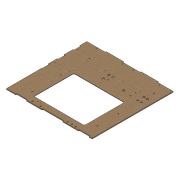
# Autodesk Inventor part: Lateral Izquierdo Carcasa
Saved by Autodesk Inventor 2020 (Build 240168000, 168)
## iProperties
Created: 2020-06-08
Part Number: Lateral Izquierdo Carcasa
Material: MDF Tablero de fibras de densidad media
Document SubType Name: Modelado
Designer: Pipi
Density: 0.8 g/cm^3
Appearance: Cartón - Ondulado
Mass: 1381.88 g
Surface Area: 4222.27 cm^2
Volume: 1727.35 cm^3
Sheet Metal Rule: Default
Author: Pipi
Autodesk Inventor part; units mm, degrees
ref_plane "YZ Plane" through (0, 0, 0) normal (1, 0, 0) x (0, 1, 0)
ref_plane "XZ Plane" through (0, 0, 0) normal (0, 1, 0) x (-1, 0, 0)
ref_plane "XY Plane" through (0, 0, 0) normal (0, 0, 1) x (1, 0, 0)
sketch "Boceto1" plane through (0, 0, 0) normal (0, 1, 0) x (-1, 0, 0)
  line L0 (67.9623, 11.1833) -> (67.9623, -453.8167)
  line L1 (435.9623, -258.8167) -> (159.9623, -258.8167)
  line L2 (152.9623, -251.8167) -> (152.9623, -35.8167)
  line L3 (159.9623, -28.8167) -> (435.9623, -28.8167)
  line L4 (442.9623, -35.8167) -> (442.9623, -251.8167)
  arc A0 (435.9623, -258.8167) -> (442.9623, -251.8167) centre (435.9623, -251.8167) ccw
  arc A1 (442.9623, -35.8167) -> (435.9623, -28.8167) centre (435.9623, -35.8167) ccw
  arc A2 (159.9623, -28.8167) -> (152.9623, -35.8167) centre (159.9623, -35.8167) ccw
  arc A3 (152.9623, -251.8167) -> (159.9623, -258.8167) centre (159.9623, -251.8167) ccw
  line L5 (449.9623, -251.8167) -> (449.9623, -35.8167)
  line L6 (435.9623, -21.8167) -> (159.9623, -21.8167)
  line L7 (145.9623, -35.8167) -> (145.9623, -251.8167)
  line L8 (159.9623, -265.8167) -> (435.9623, -265.8167)
  line L9 (159.9623, -265.8167) -> (152.9623, -265.8167)
  line L10 (145.9623, -258.8167) -> (145.9623, -251.8167)
  line L11 (159.9623, -21.8167) -> (152.9623, -21.8167)
  line L12 (145.9623, -28.8167) -> (145.9623, -35.8167)
  line L13 (435.9623, -21.8167) -> (442.9623, -21.8167)
  line L14 (449.9623, -28.8167) -> (449.9623, -35.8167)
  line L15 (449.9623, -251.8167) -> (449.9623, -258.8167)
  line L16 (442.9623, -265.8167) -> (435.9623, -265.8167)
  arc A4 (449.9623, -28.8167) -> (442.9623, -21.8167) centre (442.9623, -28.8167) ccw
  arc A5 (442.9623, -265.8167) -> (449.9623, -258.8167) centre (442.9623, -258.8167) ccw
  arc A6 (145.9623, -258.8167) -> (152.9623, -265.8167) centre (152.9623, -258.8167) ccw
  arc A7 (152.9623, -21.8167) -> (145.9623, -28.8167) centre (152.9623, -28.8167) ccw
  line L17 (557.9623, -453.8167) -> (457.9623, -453.8167)
  line L18 (457.9623, -453.8167) -> (457.9623, -459.3167)
  line L19 (457.9623, -459.3167) -> (357.9623, -459.3167)
  line L20 (357.9623, -459.3167) -> (357.9623, -453.8167)
  line L21 (357.9623, -453.8167) -> (257.9623, -453.8167)
  line L22 (257.9623, -453.8167) -> (257.9623, -459.3167)
  line L23 (257.9623, -459.3167) -> (157.9623, -459.3167)
  line L24 (157.9623, -459.3167) -> (157.9623, -453.8167)
  line L25 (157.9623, -453.8167) -> (67.9623, -453.8167)
  line L26 (157.9623, -459.3167) -> (257.9623, -459.3167)
  line L27 (357.9623, -459.3167) -> (457.9623, -459.3167)
  line L28 (355.9623, 11.1833) -> (355.9623, 5.6833)
  line L29 (355.9623, 5.6833) -> (235.9623, 5.6833)
  line L30 (235.9623, 5.6833) -> (235.9623, 11.1833)
  line L31 (67.9623, 11.1833) -> (85.9623, 11.1833)
  circle A8 centre (112.9623, -63.8167) radius 3
  circle A9 centre (112.9623, -183.8167) radius 3
  line L32 (67.9623, 11.1833) -> (85.9623, 11.1833)
  line L33 (87.9623, 5.6833) -> (87.9623, -422.8167)
  line L34 (87.9623, -422.8167) -> (137.9623, -422.8167)
  line L35 (137.9623, -422.8167) -> (137.9623, 5.6833)
  circle A10 centre (112.9623, -388.3167) radius 3
  line L36 (557.9623, 11.1833) -> (560.4623, 11.1833)
  line L37 (560.4623, 11.1833) -> (560.4623, -193.8167)
  line L38 (560.4623, -193.8167) -> (557.9623, -193.8167)
  line L39 (557.9623, -193.8167) -> (557.9623, -233.8168)
  line L40 (557.9623, -233.8168) -> (563.4623, -233.8168)
  line L41 (563.4623, -233.8168) -> (563.4623, -283.8168)
  line L42 (563.4623, -283.8168) -> (557.9623, -283.8168)
  line L43 (557.9623, -283.8168) -> (557.9623, -323.8168)
  line L44 (557.9623, -323.8168) -> (563.4623, -323.8168)
  line L45 (563.4623, -323.8168) -> (563.4623, -373.8168)
  line L46 (563.4623, -373.8168) -> (557.9623, -373.8168)
  line L47 (557.9623, -373.8168) -> (557.9623, -413.8168)
  line L48 (557.9623, -413.8168) -> (563.4623, -413.8168)
  line L49 (563.4623, -413.8168) -> (563.4623, -453.8167)
  line L50 (426.4606, 11.1833) -> (362.9606, 11.1833)
  arc A11 (376.2623, 2.6833) -> (371.2623, 2.6833) centre (373.7623, 2.6833) ccw
  arc A12 (399.7123, 1.6833) -> (394.7123, 1.6833) centre (397.2123, 1.6833) ccw
  arc A13 (424.1623, 2.6833) -> (419.1623, 2.6833) centre (421.6623, 2.6833) ccw
  line L51 (371.2623, 2.6833) -> (371.2623, -1.3167)
  line L52 (376.2623, 2.6833) -> (376.2623, -1.3167)
  arc A14 (371.2623, -1.3167) -> (376.2623, -1.3167) centre (373.7623, -1.3167) ccw
  line L53 (419.1623, 2.6833) -> (419.1623, -1.3167)
  line L54 (424.1623, 2.6833) -> (424.1623, -1.3167)
  arc A15 (419.1623, -1.3167) -> (424.1623, -1.3167) centre (421.6623, -1.3167) ccw
  line L55 (394.7123, 1.6833) -> (394.7123, -1.8167)
  line L56 (399.7123, 1.6833) -> (399.7123, -1.8167)
  arc A16 (394.7123, -1.8167) -> (399.7123, -1.8167) centre (397.2123, -1.8167) ccw
  line L57 (162.9623, 11.1833) -> (226.4623, 11.1833)
  arc A17 (221.6623, 2.6833) -> (216.6623, 2.6833) centre (219.1623, 2.6833) ccw
  arc A18 (197.2123, 1.6833) -> (192.2123, 1.6833) centre (194.7123, 1.6833) ccw
  arc A19 (173.7623, 2.6833) -> (168.7623, 2.6833) centre (171.2623, 2.6833) ccw
  line L58 (221.6623, 2.6833) -> (221.6623, -1.3167)
  line L59 (216.6623, 2.6833) -> (216.6623, -1.3167)
  arc A20 (216.6623, -1.3167) -> (221.6623, -1.3167) centre (219.1623, -1.3167) ccw
  line L60 (173.7623, 2.6833) -> (173.7623, -1.3167)
  line L61 (168.7623, 2.6833) -> (168.7623, -1.3167)
  arc A21 (168.7623, -1.3167) -> (173.7623, -1.3167) centre (171.2623, -1.3167) ccw
  line L62 (197.2123, 1.6833) -> (197.2123, -1.8167)
  line L63 (192.2123, 1.6833) -> (192.2123, -1.8167)
  arc A22 (192.2123, -1.8167) -> (197.2123, -1.8167) centre (194.7123, -1.8167) ccw
  line L64 (563.4623, -453.8167) -> (557.9623, -453.8167)
  circle A23 centre (498.4623, -445.3167) radius 2
  circle A24 centre (348.4623, -445.3167) radius 2
  circle A25 centre (137.9623, -445.3167) radius 2
  circle A26 centre (287.9623, -445.3167) radius 2
  circle A27 centre (550.2473, -388.8167) radius 2
  circle A28 centre (550.2473, -258.8167) radius 2
  circle A29 centre (77.6773, -448.8167) radius 2
  line L65 (355.9623, 11.1833) -> (445.9623, 11.1833)
  line L66 (445.9623, 11.1833) -> (445.9623, 5.6833)
  line L67 (445.9623, 5.6833) -> (505.9623, 5.6833)
  line L68 (505.9623, 5.6833) -> (505.9623, 11.1833)
  line L69 (557.9623, 11.1833) -> (505.9623, 11.1833)
  line L70 (445.9623, 11.1833) -> (355.9623, 11.1833)
  line L71 (235.9623, 11.1833) -> (145.9623, 11.1833)
  line L72 (145.9623, 11.1833) -> (145.9623, 5.6833)
  line L73 (145.9623, 5.6833) -> (85.9623, 5.6833)
  line L74 (85.9623, 5.6833) -> (85.9623, 11.1833)
  line L75 (235.9623, 11.1833) -> (145.9623, 11.1833)
  line L76 (85.9623, 11.1833) -> (67.9623, 11.1833)
  circle A30 centre (403.7123, -13.8167) radius 1.5
  circle A31 centre (390.7123, -13.8167) radius 1.5
  point P0 (145.9623, -21.8167)
  point P1 (449.9623, -21.8167)
  point P2 (449.9623, -265.8167)
  point P3 (0, 0)
  point P4 (0, 0)
  point P5 (426.4606, 11.1833)
  point P6 (362.9606, 11.1833)
  dimension "d217" = 85
  dimension "d219" = 7
  dimension "d232" = 230
  dimension "d233" = 7
  dimension "d234" = 7
  dimension "d236" = 100
  dimension "d237" = 100
  dimension "d238" = 100
  dimension "d239" = 100
  dimension "d241" = 465
  dimension "d288" = 202
  dimension "d289" = 5.5
  dimension "d292" = 168
  dimension "d312" = 6
  dimension "d314" = 6
  dimension "d319" = 120
  dimension "d325" = 50
  dimension "d326" = 25
  dimension "d327" = 25
  dimension "d328" = 6
  dimension "d329" = 25
  dimension "d332" = 34.5
  dimension "d333" = 2.5
  dimension "d334" = 205
  dimension "d336" = 27.5
  dimension "d337" = 7
  dimension "d338" = 7
  dimension "d339" = 5.5
  dimension "d342" = 40.0001
  dimension "d344" = 465
  dimension "d346" = 2.5
  dimension "d347" = 50
  dimension "d348" = 40
  dimension "d349" = 50
  dimension "d350" = 40
  dimension "d384" = 5
  dimension "d385" = 5
  dimension "d386" = 5
  dimension "d394" = 4
  dimension "d395" = 4
  dimension "d396" = 4
  dimension "d397" = 4
  dimension "d398" = 3.5
  dimension "d399" = 3.5
  dimension "d404" = 15.3
  dimension "d405" = 120
  dimension "d406" = 495.5
  dimension "d420" = 5.5
  dimension "d423" = 4
  dimension "d424" = 65
  dimension "d425" = 8.5
  dimension "d426" = 4
  dimension "d427" = 150
  dimension "d428" = 4
  dimension "d429" = 8.5
  dimension "d430" = 70
  dimension "d431" = 4
  dimension "d432" = 150
  dimension "d435" = 4
  dimension "d436" = 4
  dimension "d437" = 7.715
  dimension "d438" = 7.715
  dimension "d439" = 65
  dimension "d440" = 130
  constraints: 154 end point, 44 perpendicular, 40 point on circle, 32 centre point, 25 tangent, 19 point on line, 7 horizontal, 6 equal radius, 4 parallel, 3 collinear, 2 vertical
  measures "d217" distance between parallel lines of L0 L2
  measures "d219" radius of A0
  measures "d232" distance between parallel lines of L1 L3
  measures "d233" distance between parallel lines of L4 L5
  measures "d234" radius of A4
  measures "d236" distance of L17.start L17.end
  measures "d237" distance of L18.end L19.end
  measures "d238" distance of L20.end L21.end
  measures "d239" distance of L23.end L22.end
  measures "d241" distance of L0.start L0.end
  measures "d288" distance of L36.start L28.start
  measures "d289" distance of L28.start L28.end
  measures "d292" distance of L30.end L0.start
  measures "d312" diameter of A8
  measures "d314" diameter of A9
  measures "d319" distance of A9.centre A8.centre
  measures "d325" distance of L33.end L34.end
  measures "d326" distance from line of L35 A8.centre
  measures "d327" distance from line of L35 A9.centre
  measures "d328" diameter of A10
  measures "d329" distance from line of L35 A10.centre
  measures "d332" distance from line of L34 A10.centre
  measures "d333" distance of L36.start L36.end
  measures "d334" distance of L36.end L37.end
  measures "d336" distance between parallel lines of L29 L6
  measures "d337" distance between parallel lines of L6 L3
  measures "d338" distance between parallel lines of L1 L8
  measures "d339" distance of L17.start L49.end
  measures "d342" distance of L38.end L39.end
  measures "d344" distance from line of L36.end L17
  measures "d346" distance of L38.end L37.end
  measures "d347" distance of L40.end L41.end
  measures "d348" distance of L42.end L43.end
  measures "d349" distance of L44.end L45.end
  measures "d350" distance of L46.end L47.end
  measures "d384" diameter of A11
  measures "d385" diameter of A12
  measures "d386" diameter of A13
  measures "d394" distance of L51.start L51.end
  measures "d395" distance of L52.start L52.end
  measures "d396" distance of L53.start L53.end
  measures "d397" distance of L54.start L54.end
  measures "d398" distance of L55.start L55.end
  measures "d399" distance of L56.start L56.end
  measures "d404" distance between parallel lines of L51 L28
  measures "d405" distance of L28.end L29.end
  measures "d406" distance between parallel lines of L0 L49
  measures "d420" distance between parallel lines of L43 L41
  measures "d423" diameter of A23
  measures "d424" distance from line of L49 A23.centre
  measures "d425" distance from line of L17 A23.centre
  measures "d426" diameter of A24
  measures "d427" distance of A24.centre A23.centre
  measures "d428" diameter of A25
  measures "d429" distance from line of L25 A25.centre
  measures "d430" distance from line of L0 A25.centre
  measures "d431" diameter of A26
  measures "d432" distance of A25.centre A26.centre
  measures "d435" diameter of A27
  measures "d436" diameter of A28
  measures "d437" distance from line of L47 A27.centre
  measures "d438" distance from line of L47 A28.centre
  measures "d439" distance from line of L17 A27.centre
  measures "d440" distance of A28.centre A27.centre
extrude "Extrusión1" add sketch "Boceto1" against normal blind 5.5 contours L31 L74 L73 L33 L34 L35 L72 L71 L57 L30 L29 L28 L65 L50 L66 L67 L68 L69 L36 L37 L38 L39 L40 L41 L42 L43 L44 L45 L46 L47 L48 L49 L64 L17 L18 L19 L20 L21 L22 L23 L24 L25 L0 | L73 L35 L34 L33 | L56 A16 L55 A12
extrude "Extrusión4" add sketch "Boceto1" against normal blind 2.5 contours L15 A5 L16 L8 L9 A6 L10 L7 L12 A7 L11 L6 L13 A4 L14 L5
sketch "Boceto2" plane through (0, 0, 0) normal (0, 1, 0) x (1, 0, 0)
  line L0 (-347.4623, 291.6167) -> (-87.9623, 291.6167)
  line L1 (-87.9623, 291.6167) -> (-87.9623, 356.1167)
  line L2 (-347.4623, 291.6167) -> (-347.4623, 356.1167)
  line L3 (-347.4623, 356.1167) -> (-87.9623, 356.1167)
  line L4 (-67.9623, -11.1833) -> (-67.9623, 453.8167) projected
  circle A0 centre (-122.9623, 306.1167) radius 6
  circle A1 centre (-122.9623, 341.1167) radius 6
  circle A2 centre (-102.9623, 341.1167) radius 6
  circle A3 centre (-102.9623, 306.1167) radius 6
  circle A4 centre (-213.9623, 316.1167) radius 6
  circle A5 centre (-330.9623, 316.1167) radius 6
  line L5 (-347.4623, 356.1167) -> (-347.4623, 351.1167)
  circle A6 centre (-334.9623, 351.1167) radius 6
  circle A7 centre (-309.9623, 351.1167) radius 6
  line L6 (-435.9623, 258.8167) -> (-159.9623, 258.8167) projected
  line L7 (-257.9623, 453.8167) -> (-357.9623, 453.8167) projected
  circle A8 centre (-167.9623, 309.6167) radius 3
  circle A9 centre (-167.9623, 338.1167) radius 3
  circle A10 centre (-312.4623, 324.1167) radius 3
  point P0 (0, 0)
  point P1 (-13.9376, -9.2183)
  dimension "d130" = 259.5
  dimension "d131" = 64.5
  dimension "d132" = 20
  dimension "d134" = 12
  dimension "d135" = 12
  dimension "d136" = 12
  dimension "d137" = 12
  dimension "d140" = 20
  dimension "d141" = 15
  dimension "d144" = 20
  dimension "d145" = 15
  dimension "d146" = 12
  dimension "d147" = 12
  dimension "d150" = 126
  dimension "d151" = 243
  dimension "d157" = 12
  dimension "d158" = 12
  dimension "d227" = 35
  dimension "d228" = 35
  dimension "d297" = 6
  dimension "d298" = 6
  dimension "d300" = 6
  dimension "d301" = 80
  dimension "d302" = 80
  dimension "d303" = 18
  dimension "d304" = 18
  dimension "d307" = 32
  dimension "d308" = 35
  dimension "d340" = 32.8
  dimension "d445" = 5
  dimension "d446" = 5
  dimension "d447" = 12.5
  dimension "d448" = 37.5
  dimension "d449" = 15
  dimension "d450" = 15
  dimension "d451" = 40
  dimension "d452" = 40
  constraints: 11 centre point, 10 end point, 2 perpendicular, 1 horizontal, 1 point on line, 1 vertical, 1 other
  measures "d130" distance of L0.start L0.end
  measures "d131" distance of L0.end L1.end
  measures "d134" diameter of A0
  measures "d135" diameter of A1
  measures "d136" diameter of A2
  measures "d137" diameter of A3
  measures "d140" distance of A3.centre A0.centre
  measures "d141" distance from line of L1 A3.centre
  measures "d144" distance of A2.centre A1.centre
  measures "d145" distance from line of L1 A2.centre
  measures "d146" diameter of A4
  measures "d147" diameter of A5
  measures "d150" distance from line of L1 A4.centre
  measures "d151" distance from line of L1 A5.centre
  measures "d157" diameter of A6
  measures "d158" diameter of A7
  measures "d227" distance of A1.centre A0.centre
  measures "d228" distance of A2.centre A3.centre
  measures "d297" diameter of A8
  measures "d298" diameter of A9
  measures "d300" diameter of A10
  measures "d301" distance from line of L1 A9.centre
  measures "d302" distance from line of L1 A8.centre
  measures "d303" distance from line of L0 A8.centre
  measures "d304" distance from line of L3 A9.centre
  measures "d307" distance from line of L3 A10.centre
  measures "d308" distance from line of L2 A10.centre
  measures "d340" distance between parallel lines of L0 L6
  measures "d445" distance from line of L3 A7.centre
  measures "d446" distance from line of L3 A6.centre
  measures "d447" distance from line of L2 A6.centre
  measures "d448" distance from line of L2 A7.centre
  measures "d449" distance from line of L3 A1.centre
  measures "d450" distance from line of L3 A2.centre
  measures "d451" distance from line of L3 A4.centre
  measures "d452" distance from line of L3 A5.centre
extrude "Extrusión5" cut sketch "Boceto2" against normal blind 10 contours A7 L3 | L3 A7 | A6 L3 | L3 A6 | A0 | A1 | A2 | A3 | A4 | A5 | A8 | A9 | A10
sketch "Boceto3" plane through (0, 0, 0) normal (0, 1, 0) x (1, 0, 0)
  circle A0 centre (-471.6043, 46.8167) radius 3
  circle A1 centre (-471.6043, 211.8167) radius 3
  circle A2 centre (-471.6043, 376.8167) radius 3
  line L0 (-557.9623, 233.8168) -> (-557.9623, 193.8167) projected
  line L1 (-560.4623, -11.1833) -> (-505.9623, -11.1833) projected
  line L2 (-560.4623, 193.8167) -> (-560.4623, -11.1833) projected
  line L3 (-557.9623, 413.8168) -> (-557.9623, 373.8168) projected
  point P0 (0, 0)
  point P1 (-503.9376, 235.7818)
  point P2 (-355.9623, -11.1833)
  dimension "d207" = 6
  dimension "d208" = 6
  dimension "d209" = 6
  dimension "d352" = 165
  dimension "d353" = 165
  dimension "d354" = 58
  dimension "d355" = 88.858
  dimension "d356" = 86.358
  dimension "d357" = 86.358
  constraints: 3 centre point, 1 other
  measures "d207" diameter of A0
  measures "d208" diameter of A1
  measures "d209" diameter of A2
  measures "d352" distance of A0.centre A1.centre
  measures "d353" distance of A2.centre A1.centre
  measures "d354" distance from line of L1 A0.centre
  measures "d355" distance from line of L2 A0.centre
  measures "d357" distance from line of L3 A2.centre
extrude "Extrusión6" cut sketch "Boceto3" against normal blind 10
